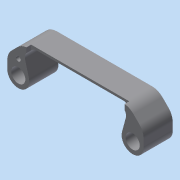
# Autodesk Inventor part: Dconnector Nutplate
Saved by Autodesk Inventor 2016 (Build 200138000, 138)
## iProperties
Created: 2016-10-07
Part Number: Dconnector Nutplate
Material: Generic
Document SubType Name: Modeling
Designer: Zara
Density: 1 g/cm^3
Appearance: Default
Author: Zara
Autodesk Inventor part; units mm, degrees
ref_plane "YZ Plane" through (0, 0, 0) normal (1, 0, 0) x (0, 1, 0)
ref_plane "XZ Plane" through (0, 0, 0) normal (0, 1, 0) x (-1, 0, 0)
ref_plane "XY Plane" through (0, 0, 0) normal (0, 0, 1) x (1, 0, 0)
sketch "Sketch1" plane through (0, 0, 0) normal (0, 0, 1) x (1, 0, 0)
  line L0 (0, 0) -> (6.3884, 0)
  line L1 (8.6334, -0.9299) -> (9.9486, -2.2451)
  arc A0 (8.6334, -0.9299) -> (6.3884, 0) centre (6.3884, -3.175) ccw
  arc A1 (10.8785, -4.4901) -> (9.9486, -2.2451) centre (7.7035, -4.4901) ccw
  line L2 (10.8785, -4.4901) -> (10.8785, -6.0198)
  arc A2 (6.1423, -5.5871) -> (10.8785, -6.0198) centre (8.4731, -6.2117) ccw
  line L3 (6.1423, -5.5871) -> (7.0336, -2.2609)
  arc A3 (7.0336, -2.2609) -> (5.4407, -0.508) centre (5.4407, -2.1082) ccw
  line L4 (5.4407, -0.508) -> (0, -0.508)
  line L5 (-4.0237, 8.5298) -> (-4.0237, -15.6063)
  line L6 (0, 0) -> (-14.4357, 0)
  line L7 (-16.6808, -0.9299) -> (-17.9959, -2.2451)
  arc A4 (-14.4357, 0) -> (-16.6808, -0.9299) centre (-14.4357, -3.175) ccw
  arc A5 (-17.9959, -2.2451) -> (-18.9258, -4.4901) centre (-15.7508, -4.4901) ccw
  line L8 (-18.9258, -4.4901) -> (-18.9258, -6.0198)
  arc A6 (-18.9258, -6.0198) -> (-14.1897, -5.5871) centre (-16.5205, -6.2117) ccw
  line L9 (-14.1897, -5.5871) -> (-15.081, -2.2609)
  arc A7 (-13.4881, -0.508) -> (-15.081, -2.2609) centre (-13.4881, -2.1082) ccw
  line L10 (-13.4881, -0.508) -> (0, -0.508)
  circle A8 centre (8.4731, -6.2117) radius 1.5494
  circle A9 centre (-16.5205, -6.2117) radius 1.5494
  point P0 (10.8785, 0)
  point P1 (7.7035, 0)
  point P2 (10.8785, -3.175)
  point P3 (-18.9258, 0)
  point P4 (-15.7508, 0)
  point P5 (-18.9258, -3.175)
  dimension "d7" = 3.175
  dimension "d8" = 3.175
  dimension "d9" = 3.175
  dimension "d10" = 3.175
  dimension "d11" = 6.0198
  dimension "d12" = 2.413
  dimension "d13" = 1.6002
  dimension "d14" = 0.508
  dimension "d15" = 75
  dimension "d16" = 24.9936
  dimension "d19" = 3.0988
  dimension "d20" = 3.0988
  constraints: 22 end point, 16 point on circle, 15 symmetric about line, 10 centre point, 8 point on line, 5 tangent, 2 coincident, 2 horizontal, 2 vertical, 4 other
  measures "d7" distance of point (7.703, 0) point (10.878, 0)
  measures "d8" distance of point (10.878, -3.175) point (10.878, 0)
  measures "d9" radius of A0
  measures "d10" radius of A1
  measures "d11" distance from line of L2.end L0
  measures "d12" radius of A2
  measures "d13" radius of A3
  measures "d14" distance between parallel lines of L0 L4
  measures "d15" angle of L3 L4
  measures "d16" distance of A2.centre A6.centre
  measures "d19" diameter of A8
  measures "d20" diameter of A9
extrude "Extrusion2" add sketch "Sketch1" along normal blind 5.334
sketch "Sketch4" plane through (0, 0, 5.334) normal (0, 0, 1) x (1, 0, 0)
  circle A0 centre (-16.5205, -6.2117) radius 1.5494 projected
  circle A1 centre (8.4731, -6.2117) radius 1.5494 projected
  line L0 (6.3884, 0) -> (-14.4357, 0) projected
  arc A2 (-14.4357, 0) -> (-16.6808, -0.9299) centre (-14.4357, -3.175) ccw projected
  line L1 (-16.6808, -0.9299) -> (-17.9959, -2.2451) projected
  arc A3 (-17.9959, -2.2451) -> (-18.9258, -4.4901) centre (-15.7508, -4.4901) ccw projected
  line L2 (-18.9258, -4.4901) -> (-18.9258, -6.0198) projected
  arc A4 (-18.9258, -6.0198) -> (-14.1897, -5.5871) centre (-16.5205, -6.2117) ccw projected
  line L3 (-14.1897, -5.5871) -> (-15.081, -2.2609) projected
  arc A5 (-13.4881, -0.508) -> (-15.081, -2.2609) centre (-13.4881, -2.1082) ccw projected
  line L4 (-13.4881, -0.508) -> (5.4407, -0.508) projected
  arc A6 (7.0336, -2.2609) -> (5.4407, -0.508) centre (5.4407, -2.1082) ccw projected
  line L5 (7.0336, -2.2609) -> (6.1423, -5.5871) projected
  arc A7 (6.1423, -5.5871) -> (10.8785, -6.0198) centre (8.4731, -6.2117) ccw projected
  line L6 (10.8785, -6.0198) -> (10.8785, -4.4901) projected
  arc A8 (10.8785, -4.4901) -> (9.9486, -2.2451) centre (7.7035, -4.4901) ccw projected
  line L7 (9.9486, -2.2451) -> (8.6334, -0.9299) projected
  arc A9 (8.6334, -0.9299) -> (6.3884, 0) centre (6.3884, -3.175) ccw projected
  line L8 (6.6951, 0.8344) -> (6.6951, -4.1165) construction
  line L9 (6.6951, -0.0149) -> (6.6951, -1.1147)
  line L10 (-14.7425, 1.6271) -> (-14.7425, -3.2751) construction
  line L11 (-14.7425, -0.0149) -> (-14.7425, -1.1147)
  point P0 (0, 0)
  dimension "d24" = 1.778
  dimension "d25" = 1.778
  constraints: 8 end point, 4 point on circle, 4 point on line, 2 vertical
  measures "d24" distance from line of L8 A1.centre
  measures "d25" distance from line of A0.centre L10
extrude "Extrusion3" add sketch "Sketch4" along normal blind 1.016 contours A9 L7 A8 L6 A7 L5 A6 L9 | L11 A5 L3 A4 L2 A3 L1 A2
sketch "Sketch5" plane through (0, 0, 6.35) normal (0, 0, 1) x (1, 0, 0)
  circle A0 centre (-16.5205, -6.2117) radius 1.5494 projected
  line L0 (-16.6808, -0.9299) -> (-17.9959, -2.2451) projected
  arc A1 (-17.9959, -2.2451) -> (-18.9258, -4.4901) centre (-15.7508, -4.4901) ccw projected
  line L1 (-18.9258, -4.4901) -> (-18.9258, -6.0198) projected
  arc A2 (-18.9258, -6.0198) -> (-14.1897, -5.5871) centre (-16.5205, -6.2117) ccw projected
  line L2 (-14.1897, -5.5871) -> (-15.081, -2.2609) projected
  arc A3 (-14.7425, -1.1147) -> (-15.081, -2.2609) centre (-13.4881, -2.1082) ccw projected
  line L3 (-14.7425, -1.1147) -> (-14.7425, -0.0149) projected
  arc A4 (-14.7425, -0.0149) -> (-16.6808, -0.9299) centre (-14.4357, -3.175) ccw projected
  circle A5 centre (-16.5205, -3.048) radius 0.5207
  line L4 (6.3884, 0) -> (-14.4357, 0) projected
  point P0 (0, 0)
  dimension "d28" = 3.048
  dimension "d29" = 1.0414
  constraints: 1 centre point
  measures "d28" distance from line of L4 A5.centre
  measures "d29" diameter of A5
extrude "Extrusion4" cut sketch "Sketch5" against normal blind 1.27 contours A5
equation "\"d8\" = d7"
body "Solid2"
